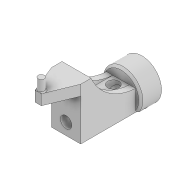
# Autodesk Inventor part: Cart
Saved by Autodesk Inventor 2020 (Build 240168000, 168)
## iProperties
Created: 2022-06-17
Part Number: Cart
Material: Generic
Document SubType Name: Modeling
Designer: ferrerx
Density: 1 g/cm^3
Appearance: Default
Author: ferrerx
Autodesk Inventor part; units mm, degrees
ref_plane "YZ Plane" through (0, 0, 0) normal (1, 0, 0) x (0, 1, 0)
ref_plane "XZ Plane" through (0, 0, 0) normal (0, 1, 0) x (-1, 0, 0)
ref_plane "XY Plane" through (0, 0, 0) normal (0, 0, 1) x (1, 0, 0)
sketch "Sketch1" plane through (0, 0, 0) normal (0, 1, 0) x (-1, 0, 0)
  line L0 (-7, 16.25) -> (7, 16.25)
  line L1 (7, 16.25) -> (7, -16.25)
  line L2 (7, -16.25) -> (-7, -16.25)
  line L3 (-7, -16.25) -> (-7, 16.25)
  line L4 (-7, 16.25) -> (7, -16.25) construction
  line L5 (7, 16.25) -> (-7, -16.25) construction
  circle A0 centre (0, 12.5) radius 1.3
  line L6 (0, 12.5) -> (0, -2.5) construction
  circle A1 centre (0, -2.5) radius 1.3
  point P0 (0, 0)
  dimension "d0" = 14
  dimension "d1" = 32.5
  dimension "d2" = 2.6
  dimension "d3" = 15
  dimension "d4" = 2.6
  dimension "d5" = 12.5
  constraints: 14 end point, 2 centre point, 2 midpoint, 2 parallel, 1 coincident, 1 horizontal, 1 perpendicular, 1 vertical
  measures "d0" distance of L1.end L2.end
  measures "d1" distance of L2.end L0.start
  measures "d2" diameter of A1
  measures "d3" distance of L6.start L6.end
  measures "d4" diameter of A0
  measures "d5" distance of point (0, 0) L6.start
extrude "Extrusion1" add sketch "Sketch1" along normal blind 10
sketch "Sketch2" plane through (7, 0, -16.25) normal (0, 0, -1) x (-1, 0, 0)
  line L0 (7, 0) -> (7, 10) construction
  circle A0 centre (7, 5.666) radius 4
  line L1 (0, 0) -> (14, 0) projected
  dimension "d8" = 5.666
  dimension "d9" = 8
  constraints: 2 end point, 1 centre point, 1 point on line, 1 vertical
  measures "d8" distance from line of L1 A0.centre
  measures "d9" diameter of A0
extrude "Extrusion2" cut sketch "Sketch2" against normal blind 6.5
sketch "Sketch3" plane through (0, 5.666, -9.75) normal (0, 0, -1) x (-1, 0, 0)
  circle A0 centre (0, 0) radius 2.75
  circle A1 centre (0, 0) radius 4 projected
  point P0 (0, -5.666)
  dimension "d12" = 5.5
  constraints: 1 centre point, 1 concentric
  measures "d12" diameter of A0
extrude "Extrusion3" cut sketch "Sketch3" against normal blind 42.25 contours A0
sketch "Sketch4" plane through (7, 0, -16.25) normal (0, 0, -1) x (-1, 0, 0)
  circle A0 centre (7, 5.666) radius 4 projected
  circle A1 centre (7, 5.666) radius 9.5
  line L0 (-0.6254, 0) -> (14.6254, 0)
  point P0 (7, 0)
  dimension "d15" = 19
  constraints: 2 end point, 2 point on circle, 1 centre point, 1 coincident, 1 horizontal
  measures "d15" diameter of A1
extrude "Extrusion4" add sketch "Sketch4" against normal blind 10 contours A1 L0 picked at (7.1607, 0.5651)
sketch "Sketch7" plane through (0, 5.666, -16.25) normal (0, 0, -1) x (-1, 0, 0)
  circle A0 centre (0, 0) radius 9.5
  circle A1 centre (0, 0) radius 4 projected
  line L0 (-7.6254, -5.666) -> (7.6254, -5.666) projected
  line L1 (-7.6254, -5.666) -> (7.6254, -5.666)
  point P0 (0, -5.666)
  constraints: 2 end point, 1 centre point, 1 collinear, 1 point on circle
extrude "Extrusion7" add sketch "Sketch7" against normal blind 4.8 contours L0 A0 picked at (-2.0372, -6.2017)
sketch "Sketch5" plane through (0, 10, 0) normal (0, 1, 0) x (1, 0, 0)
  circle A0 centre (0, -12.5) radius 1.3 projected
  circle A1 centre (0, -12.5) radius 2.75
  circle A2 centre (0, 2.5) radius 1.3 projected
  circle A3 centre (0, 2.5) radius 2.75
  point P0 (0, 0)
  dimension "d18" = 5.5
  dimension "d19" = 5.5
  constraints: 2 centre point, 2 coincident
  measures "d18" diameter of A1
  measures "d19" diameter of A3
extrude "Extrusion5" cut sketch "Sketch5" against normal blind 7.5 contours A0 | A1 | A2 | A3
chamfer "Chamfer1" distance 1.2 angle 45 2 edges at (1.3, 2.5, 12.5) (1.3, 2.5, -2.5)
sketch "Sketch6" plane through (0, 5.666, -16.25) normal (0, 0, -1) x (-1, 0, 0)
  circle A0 centre (0, 0) radius 6.35 construction
  line L0 (0, 0) -> (-5.4993, 3.175) construction
  circle A1 centre (-5.4993, 3.175) radius 2
  line L1 (0, 0) -> (0, 6.35) construction
  circle A2 centre (5.4993, 3.175) radius 2
  circle A3 centre (0, -6.35) radius 2
  point P0 (0, -5.666)
  dimension "d25" = 12.7
  dimension "d26" = 60
  dimension "d27" = 4
  dimension "d30" = 4
  constraints: 4 centre point, 4 end point, 3 point on circle, 1 coincident, 1 symmetric about line, 1 vertical, 1 other
  measures "d25" diameter of A0
  measures "d26" angle of L1 L0
  measures "d27" diameter of A1
  measures "d30" diameter of A3
extrude "Extrusion6" cut sketch "Sketch6" against normal blind 5.5
fillet "Fillet1" [suppressed]
chamfer "Chamfer2" distance 1 angle 45 1 edges at (0, 15.166, -6.25)
fillet "Fillet2" [suppressed]
thicken "Thicken1" operation add thickness 4 both sides no extend neighbours yes toward (0, 0, 1) faces at (5.5833, 5.222, 16.25)
sketch "Sketch8" plane through (0, 10, 0) normal (0, 1, 0) x (1, 0, 0)
  line L0 (-7, -20.25) -> (7, -20.25) projected
  line L1 (-7, 6.25) -> (-7, -20.25) projected
  line L2 (7, -20.25) -> (-7, -20.25)
  line L3 (-7, -20.25) -> (-7, -15.25)
  line L4 (-7, -15.25) -> (7, -15.25)
  line L5 (7, -15.25) -> (7, -20.25)
  point P0 (0, 0)
  dimension "d40" = 5
  constraints: 8 end point, 2 parallel, 1 horizontal, 1 perpendicular, 1 point on line
  measures "d40" distance between parallel lines of L0 L4
extrude "Extrusion8" add sketch "Sketch8" along normal blind 15
sketch "Sketch9" plane through (7, 0.8442, -6.25) normal (1, 0, 0) x (0, 0, -1)
  line L0 (-26.5, 24.1558) -> (-21.5, 24.1558) projected
  line L1 (-21.5, 9.1558) -> (0, 9.1558) projected
  line L2 (-21.5, 24.1558) -> (0, 9.1558)
  line L3 (0, 9.1558) -> (-21.5, 9.1558)
  line L4 (-21.5, 9.1558) -> (-21.5, 24.1558) projected
  line L5 (-21.5, 9.1558) -> (-21.5, 24.1558)
  point P0 (-6.25, -0.8442)
  constraints: 6 end point, 1 collinear, 1 perpendicular
extrude "Extrusion9" add sketch "Sketch9" against normal blind 3
mirror "Mirror1" about plane through (0, 0, 0) normal (1, 0, 0) of "Extrusion9"
sketch "Sketch10" plane through (-7, 0, 20.25) normal (0, 0, 1) x (1, 0, 0)
  line L0 (14, 0) -> (14, 25) projected
  line L1 (0, 25) -> (14, 25)
  line L2 (14, 25) -> (14, 20)
  line L3 (14, 20) -> (0, 20)
  line L4 (0, 20) -> (0, 25)
  line L5 (0, 25) -> (14, 25) projected
  point P0 (7, 0)
  dimension "d45" = 5
  constraints: 8 end point, 2 parallel, 1 collinear, 1 horizontal, 1 perpendicular, 1 point on line
  measures "d45" distance between parallel lines of L1 L3
extrude "Extrusion10" add sketch "Sketch10" along normal blind 13.5
sketch "Sketch11" plane through (-7, 20, 20.25) normal (0, -1, 0) x (1, 0, 0)
  line L0 (14, 0) -> (8.5, 13.5)
  line L1 (14, 13.5) -> (0, 13.5) projected
  line L2 (8.5, 13.5) -> (14, 13.5)
  line L3 (14, 0) -> (14, -27.0058) projected
  line L4 (14, 13.5) -> (14, 0)
  line L5 (0, 0) -> (14, 0) projected
  line L6 (7, 0) -> (7, 13.5) construction
  line L7 (0, 0) -> (5.5, 13.5)
  line L8 (5.5, 13.5) -> (0, 13.5)
  line L9 (0, 13.5) -> (0, 0)
  point P0 (7, -20.25)
  dimension "d51" = 3
  constraints: 14 end point, 2 midpoint, 1 collinear, 1 perpendicular, 1 symmetric about line
  measures "d51" distance of L0.end L7.end
extrude "Extrusion11" cut sketch "Sketch11" against normal blind 10 contours L0 L1 L4 | L9 L1 L7
sketch "Sketch12" plane through (0, 25, 0) normal (0, 1, 0) x (1, 0, 0)
  circle A0 centre (0, -32.25) radius 1.5
  line L0 (1.5, -33.75) -> (-1.5, -33.75) projected
  point P0 (0, 0)
  dimension "d54" = 3
  dimension "d55" = 1.5
  constraints: 1 centre point
  measures "d54" diameter of A0
  measures "d55" distance from line of L0 A0.centre
extrude "Extrusion12" add sketch "Sketch12" along normal blind 5.5
fillet "Fillet3" radius 0.5 2 edges at (-1.0607, 25, 31.1893) (1.0607, 25, 33.3107)
sketch "Sketch13" plane through (7, 0, 20.25) normal (1, 0, 0) x (0, 0, -1)
  line L0 (5, 25) -> (5, 10) projected
  line L1 (26.5, 0.8442) -> (26.5, 10) projected
  arc A0 (5, 25) -> (26.5, 10) centre (27.9307, 34.959) ccw
  line L2 (5, 25) -> (26.5, 10)
  line L3 (26.5, 10) -> (5, 25) projected
  point P0 (20.25, 0)
  dimension "d59" = 25
  constraints: 3 point on circle, 2 end point, 1 centre point, 1 collinear
  measures "d59" radius of A0
extrude "Extrusion13" cut sketch "Sketch13" against normal blind 20
body "Solid1"
